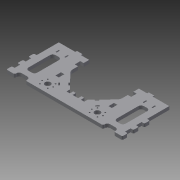
# Autodesk Inventor part: Bulkhead 27021014
Saved by Autodesk Inventor 2015 (Build 190159000, 159)
## iProperties
Created: 2014-06-30
Part Number: Bulkhead 27021014
Material: Generic
Document SubType Name: Modeling
Designer: STACKPOLE
Density: 1 g/cm^3
Appearance: Default
Author: STACKPOLE
Autodesk Inventor part; units mm, degrees
ref_plane "YZ Plane" through (0, 0, 0) normal (1, 0, 0) x (0, 1, 0)
ref_plane "XZ Plane" through (0, 0, 0) normal (0, 1, 0) x (-1, 0, 0)
ref_plane "XY Plane" through (0, 0, 0) normal (0, 0, 1) x (1, 0, 0)
sketch "Sketch1" plane through (0, 0, 0) normal (0, 0, 1) x (1, 0, 0)
  line L0 (0, -90) -> (-103, -90)
  line L1 (0, 0) -> (0, -90) construction
  line L2 (-105, -88) -> (-105, -82)
  line L3 (-103, -80) -> (-100, -80)
  line L4 (-100, -70) -> (-103, -70)
  line L5 (-105, -68) -> (-105, -62)
  line L6 (-103, -60) -> (-100, -60)
  line L7 (-100, -80) -> (-100, -70)
  line L8 (-100, -50) -> (-103, -50)
  line L9 (-105, -48) -> (-105, -42)
  line L10 (-103, -40) -> (-100, -40)
  line L11 (-100, -60) -> (-100, -50)
  line L12 (-100, -40) -> (-100, 0)
  line L13 (-70, 0) -> (-70, 3)
  line L14 (-70, 3) -> (-60, 3)
  line L15 (-60, 3) -> (-60, 0)
  line L16 (-100, 0) -> (-70, 0)
  line L17 (-60, 0) -> (-45, 0)
  line L18 (-45, 0) -> (-45, -29.9568)
  arc A0 (-105, -88) -> (-103, -90) centre (-103, -88) ccw
  arc A1 (-103, -80) -> (-105, -82) centre (-103, -82) ccw
  arc A2 (-105, -68) -> (-103, -70) centre (-103, -68) ccw
  arc A3 (-103, -60) -> (-105, -62) centre (-103, -62) ccw
  arc A4 (-105, -48) -> (-103, -50) centre (-103, -48) ccw
  arc A5 (-103, -40) -> (-105, -42) centre (-103, -42) ccw
  line L19 (0, -90) -> (103, -90)
  line L20 (105, -88) -> (105, -82)
  line L21 (103, -80) -> (100, -80)
  line L22 (100, -70) -> (103, -70)
  line L23 (105, -68) -> (105, -62)
  line L24 (103, -60) -> (100, -60)
  line L25 (100, -80) -> (100, -70)
  line L26 (100, -50) -> (103, -50)
  line L27 (105, -48) -> (105, -42)
  line L28 (103, -40) -> (100, -40)
  line L29 (100, -60) -> (100, -50)
  line L30 (100, -40) -> (100, 0)
  line L31 (70, 0) -> (70, 3)
  line L32 (70, 3) -> (60, 3)
  line L33 (60, 3) -> (60, 0)
  line L34 (100, 0) -> (70, 0)
  line L35 (60, 0) -> (45, 0)
  line L36 (45, 0) -> (45, -29.9568)
  arc A6 (103, -90) -> (105, -88) centre (103, -88) ccw
  arc A7 (105, -82) -> (103, -80) centre (103, -82) ccw
  arc A8 (103, -70) -> (105, -68) centre (103, -68) ccw
  arc A9 (105, -62) -> (103, -60) centre (103, -62) ccw
  arc A10 (103, -50) -> (105, -48) centre (103, -48) ccw
  arc A11 (105, -42) -> (103, -40) centre (103, -42) ccw
  line L37 (-42.1899, -36.907) -> (-16, -64)
  line L38 (16, -64) -> (42.1899, -36.907)
  line L39 (-16, -70) -> (-10, -70)
  line L40 (-10, -70) -> (-10, -64)
  line L41 (-5, -64) -> (-5, -70)
  line L42 (-5, -70) -> (5, -70)
  line L43 (5, -70) -> (5, -64)
  line L44 (10, -64) -> (10, -70)
  line L45 (10, -70) -> (16, -70)
  line L46 (-10, -64) -> (-5, -64)
  line L47 (5, -64) -> (10, -64)
  line L48 (16, -64) -> (16, -70)
  line L49 (-16, -64) -> (-16, -70)
  arc A12 (-45, -29.9568) -> (-42.1899, -36.907) centre (-35, -29.9568) ccw
  arc A13 (42.1899, -36.907) -> (45, -29.9568) centre (35, -29.9568) ccw
  point P0 (-105, -90)
  point P1 (-105, -80)
  point P2 (-105, -70)
  point P3 (-105, -60)
  point P4 (-105, -50)
  point P5 (-105, -40)
  point P6 (105, -90)
  point P7 (105, -80)
  point P8 (105, -70)
  point P9 (105, -60)
  point P10 (105, -50)
  point P11 (105, -40)
  point P12 (-45, -34)
  point P13 (45, -34)
  point P14 (0, -70)
  dimension "d4" = 105
  dimension "d5" = 10
  dimension "d6" = 5
  dimension "d8" = 10
  dimension "d9" = 10
  dimension "d10" = 10
  dimension "d11" = 10
  dimension "d12" = 30
  dimension "d13" = 10
  dimension "d14" = 3
  dimension "d15" = 90
  dimension "d18" = 15
  dimension "d19" = 34
  dimension "d20" = 2
  dimension "d102" = 5
  dimension "d104" = 5
  dimension "d105" = 10
  dimension "d160" = 6
  dimension "d161" = 6
  dimension "d162" = 6
  dimension "d163" = 70
  dimension "d175" = 10
  constraints: 100 end point, 36 symmetric about line, 28 point on circle, 28 point on line, 23 perpendicular, 16 tangent, 14 centre point, 10 parallel, 6 equal radius, 6 horizontal alignment, 5 vertical alignment, 2 horizontal, 1 midpoint, 1 vertical, 6 other
  measures "d4" distance of L0.start point (-105, -90)
  measures "d5" distance of point (-105, -90) point (-105, -80)
  measures "d6" distance of point (-105, -80) L3.end
  measures "d8" distance between parallel lines of L3 L4
  measures "d9" distance of point (-105, -70) point (-105, -60)
  measures "d10" distance between parallel lines of L6 L8
  measures "d11" distance of point (-105, -50) point (-105, -40)
  measures "d12" distance from line of L12 L13.start
  measures "d13" distance of L13.end L14.end
  measures "d14" distance of L13.start L13.end
  measures "d15" distance between parallel lines of L16 L0
  measures "d18" distance of L15.end L17.end
  measures "d19" distance of point (-45, -34) L17.end
  measures "d20" radius of A0
  measures "d102" distance between parallel lines of L41 L40
  measures "d104" distance between parallel lines of L44 L43
  measures "d105" distance between parallel lines of L41 L43
  measures "d160" distance of L37.end L39.start
  measures "d161" distance of L39.start L39.end
  measures "d162" distance of L44.end L45.end
  measures "d163" distance between parallel lines of L35 L42
  measures "d175" radius of A12
extrude "Extrusion1" add sketch "Sketch1" along normal blind 6
sketch "Sketch2" plane through (0, 0, 6) normal (0, 0, 1) x (1, 0, 0)
  line L0 (-103, -90) -> (103, -90) projected
  line L1 (-70, 0) -> (-100, 0) projected
  circle A0 centre (-45, -75) radius 5
  circle A1 centre (-45, -75) radius 10 construction
  line L2 (-45, -75) -> (-52.0711, -67.9289) construction
  line L3 (-45, -75) -> (-55, -75) construction
  line L4 (-55, -75) -> (-45, -75) construction
  circle A2 centre (-52.0711, -67.9289) radius 1.25
  circle A3 centre (-55, -75) radius 1.25
  circle A4 centre (-52.0711, -82.0711) radius 1.25
  line L5 (-45, -65) -> (-45, -85) construction
  circle A5 centre (-37.9289, -67.9289) radius 1.25
  circle A6 centre (-35, -75) radius 1.25
  circle A7 centre (-37.9289, -82.0711) radius 1.25
  line L6 (0, 0) -> (0, -90) construction
  circle A8 centre (45, -75) radius 5
  circle A9 centre (45, -75) radius 10 construction
  line L7 (45, -75) -> (52.0711, -67.9289) construction
  line L8 (45, -75) -> (55, -75) construction
  line L9 (55, -75) -> (45, -75) construction
  circle A10 centre (52.0711, -67.9289) radius 1.25
  circle A11 centre (55, -75) radius 1.25
  circle A12 centre (52.0711, -82.0711) radius 1.25
  line L10 (45, -65) -> (45, -85) construction
  circle A13 centre (37.9289, -67.9289) radius 1.25
  circle A14 centre (35, -75) radius 1.25
  circle A15 centre (37.9289, -82.0711) radius 1.25
  dimension "d23" = 10
  dimension "d25" = 75
  dimension "d26" = 45
  dimension "d27" = 20
  dimension "d28" = 45
  dimension "d29" = 2.5
  dimension "d30" = 2.5
  constraints: 18 end point, 16 centre point, 16 symmetric about line, 8 point on circle, 6 coincident, 1 collinear, 1 midpoint, 1 parallel, 1 perpendicular, 12 other
  measures "d23" diameter of A0
  measures "d25" vertical distance of A0.centre L6.start
  measures "d26" horizontal distance of L6.start A0.centre
  measures "d27" diameter of A1
  measures "d28" angle of L4 L2
  measures "d29" diameter of A2
  measures "d30" diameter of A3
extrude "Extrusion2" cut sketch "Sketch2" against normal blind 6
sketch "Sketch5" plane through (0, 0, 6) normal (0, 0, 1) x (1, 0, 0)
  line L0 (-83, -23) -> (-77, -23)
  line L1 (-72, -28) -> (-72, -67)
  line L2 (-77, -72) -> (-83, -72)
  line L3 (-88, -67) -> (-88, -28)
  line L4 (0, 0) -> (0, -90) construction
  line L5 (83, -23) -> (77, -23)
  line L6 (72, -28) -> (72, -67)
  line L7 (77, -72) -> (83, -72)
  line L8 (88, -67) -> (88, -28)
  arc A0 (-83, -23) -> (-88, -28) centre (-83, -28) ccw
  arc A1 (-72, -28) -> (-77, -23) centre (-77, -28) ccw
  arc A2 (-77, -72) -> (-72, -67) centre (-77, -67) ccw
  arc A3 (-88, -67) -> (-83, -72) centre (-83, -67) ccw
  arc A4 (77, -23) -> (72, -28) centre (77, -28) ccw
  arc A5 (88, -28) -> (83, -23) centre (83, -28) ccw
  arc A6 (83, -72) -> (88, -67) centre (83, -67) ccw
  arc A7 (72, -67) -> (77, -72) centre (77, -67) ccw
  line L9 (-70, 0) -> (-100, 0) projected
  line L10 (-100, 0) -> (-100, -40) projected
  line L11 (-103, -90) -> (103, -90) projected
  point P0 (-88, -23)
  point P1 (-72, -72)
  point P2 (-72, -23)
  point P3 (-88, -72)
  point P4 (88, -23)
  point P5 (72, -72)
  point P6 (72, -23)
  point P7 (88, -72)
  dimension "d65" = 5
  dimension "d187" = 23
  dimension "d188" = 12
  dimension "d189" = 16
  dimension "d190" = 18
  constraints: 18 end point, 16 point on circle, 16 point on line, 16 tangent, 8 centre point, 7 equal radius, 4 symmetric about line, 3 parallel, 1 horizontal, 1 perpendicular
  measures "d65" radius of A0
  measures "d187" distance between parallel lines of L9 L0
  measures "d188" distance between parallel lines of L10 L3
  measures "d189" distance between parallel lines of L1 L3
  measures "d190" distance between parallel lines of L11 L2
extrude "Extrusion5" cut sketch "Sketch5" against normal blind 6
sketch "Sketch3" plane through (0, 0, 6) normal (0, 0, 1) x (1, 0, 0)
  line L0 (-103, -90) -> (103, -90) projected
  line L1 (-70, 0) -> (-100, 0) projected
  line L2 (-88, -12) -> (-86, -12)
  line L3 (-86, -12) -> (-86, -18)
  line L4 (-86, -18) -> (-88, -18)
  line L5 (-88, -18) -> (-88, -12)
  line L6 (-72, -12) -> (-70, -12)
  line L7 (-70, -12) -> (-70, -18)
  line L8 (-70, -18) -> (-72, -18)
  line L9 (-72, -18) -> (-72, -12)
  line L10 (0, 0) -> (0, -90) construction
  line L11 (88, -12) -> (86, -12)
  line L12 (86, -12) -> (86, -18)
  line L13 (86, -18) -> (88, -18)
  line L14 (88, -18) -> (88, -12)
  line L15 (72, -12) -> (70, -12)
  line L16 (70, -12) -> (70, -18)
  line L17 (70, -18) -> (72, -18)
  line L18 (72, -18) -> (72, -12)
  line L19 (-100, 0) -> (-100, -40) projected
  circle A0 centre (-45, -75) radius 5 projected
  line L20 (-16, -64) -> (-42.1899, -36.907) projected
  line L21 (-45, -75) -> (-24.5118, -55.1947) construction
  line L22 (-26.5968, -53.0378) -> (-28.0348, -54.4278)
  line L23 (-28.0348, -54.4278) -> (-23.8647, -58.7417)
  line L24 (-23.8647, -58.7417) -> (-22.4267, -57.3517)
  line L25 (-26.5968, -53.0378) -> (-22.4267, -57.3517)
  line L26 (26.5968, -53.0378) -> (28.0348, -54.4278)
  line L27 (28.0348, -54.4278) -> (23.8647, -58.7417)
  line L28 (23.8647, -58.7417) -> (22.4267, -57.3517)
  line L29 (26.5968, -53.0378) -> (22.4267, -57.3517)
  line L30 (-37.3817, -63.4631) -> (-33.2115, -67.777)
  line L31 (-33.2115, -67.777) -> (-31.7736, -66.387)
  line L32 (-31.7736, -66.387) -> (-35.9437, -62.073)
  line L33 (-35.9437, -62.073) -> (-37.3817, -63.4631)
  line L34 (37.3817, -63.4631) -> (33.2115, -67.777)
  line L35 (33.2115, -67.777) -> (31.7736, -66.387)
  line L36 (31.7736, -66.387) -> (35.9437, -62.073)
  line L37 (35.9437, -62.073) -> (37.3817, -63.4631)
  point P0 (-45, -34)
  dimension "d41" = 6
  dimension "d43" = 12
  dimension "d129" = 12
  dimension "d130" = 14
  dimension "d131" = 2
  dimension "d132" = 2
  dimension "d165" = 3
  dimension "d166" = 3
  dimension "d167" = 2
  dimension "d168" = 11
  dimension "d170" = 2
  dimension "d171" = 3
  dimension "d172" = 3
  constraints: 68 end point, 16 symmetric about line, 7 parallel, 7 perpendicular, 3 point on line, 2 horizontal, 2 horizontal alignment, 1 collinear, 1 midpoint
  measures "d41" distance of L4.end L2.start
  measures "d43" distance between parallel lines of L1 L2
  measures "d129" distance between parallel lines of L5 L19
  measures "d130" distance between parallel lines of L9 L3
  measures "d131" distance of L6.start L6.end
  measures "d132" distance of L2.start L2.end
  measures "d165" distance between parallel lines of L22 L21
  measures "d166" distance between parallel lines of L24 L21
  measures "d167" distance of L22.start L22.end
  measures "d168" distance between parallel lines of L32 L23
  measures "d170" distance of L32.end L30.start
  measures "d171" distance between parallel lines of L33 L21
  measures "d172" distance between parallel lines of L31 L21
sketch "Sketch7" plane through (0, 0, 6) normal (0, 0, 1) x (1, 0, 0)
  line L0 (-100, -70) -> (-100, -80) projected
  line L1 (-103, -90) -> (103, -90) projected
  line L2 (100, -80) -> (100, -70) projected
  line L3 (-90, -90) -> (-70, -90)
  line L4 (-70, -90) -> (-70, -82)
  line L5 (-70, -82) -> (-90, -82)
  line L6 (-90, -82) -> (-90, -90)
  line L7 (90, -90) -> (70, -90)
  line L8 (70, -90) -> (70, -82)
  line L9 (70, -82) -> (90, -82)
  line L10 (90, -82) -> (90, -90)
  point P0 (0, 0)
  dimension "d135" = 10
  dimension "d136" = 8
  dimension "d137" = 20
  dimension "d138" = 10
  dimension "d139" = 20
  dimension "d140" = 8
  constraints: 16 end point, 4 parallel, 2 horizontal, 2 perpendicular, 2 point on line
  measures "d135" distance between parallel lines of L0 L6
  measures "d136" distance of L5.end L3.start
  measures "d137" distance of L4.end L5.end
  measures "d138" distance between parallel lines of L2 L10
  measures "d139" distance of L8.end L9.end
  measures "d140" distance of L9.end L7.start
extrude "Extrusion13" cut sketch "Sketch7" against normal through all
fillet "Fillet4" radius 5 4 edges at (-90, -82, 3) (-70, -82, 3) (70, -82, 3) (90, -82, 3)
fillet "Fillet5" radius 2 4 edges at (-90, -90, 3) (-70, -90, 3) (70, -90, 3) (90, -90, 3)
extrude "Extrusion15" cut sketch "Sketch3" against normal through all contours L2 L3 L4 L5 | L6 L7 L8 L9 | L14 L13 L12 L11 | L18 L17 L16 L15 | L24 L23 L22 L20 | L26 L27 L28 L29 | L33 L32 L31 L30 | L34 L35 L36 L37
fillet "Fillet7" radius 0.5 8 edges at (-26.5968, -53.0378, 3) (-28.0348, -54.4278, 3) (-23.8647, -58.7417, 3) (-22.4267, -57.3517, 3) (26.5968, -53.0378, 3) (28.0348, -54.4278, 3) (23.8647, -58.7417, 3) (22.4267, -57.3517, 3)
sketch "Sketch8" plane through (0, 0, 6) normal (0, 0, 1) x (1, 0, 0)
  line L0 (-45, -29.9568) -> (-45, 0) projected
  line L1 (-45, -10) -> (-51, -10)
  line L2 (-51, -10) -> (-51, -20)
  line L3 (-51, -20) -> (-45, -20)
  line L4 (-45, -20) -> (-45, -10)
  line L5 (-45, 0) -> (-60, 0) projected
  line L6 (-45, -45) -> (-51, -45)
  line L7 (-51, -45) -> (-51, -55)
  line L8 (-51, -55) -> (-45, -55)
  line L9 (-45, -55) -> (-45, -45)
  line L10 (45, 0) -> (45, -29.9568) projected
  line L11 (45, -10) -> (51, -10)
  line L12 (51, -10) -> (51, -20)
  line L13 (51, -20) -> (45, -20)
  line L14 (45, -20) -> (45, -10)
  line L15 (45, -45) -> (51, -45)
  line L16 (51, -45) -> (51, -55)
  line L17 (51, -55) -> (45, -55)
  line L18 (45, -55) -> (45, -45)
  point P0 (0, 0)
  dimension "d177" = 6
  dimension "d178" = 10
  dimension "d179" = 10
  dimension "d180" = 10
  dimension "d181" = 6
  dimension "d182" = 55
  dimension "d183" = 6
  dimension "d184" = 10
  constraints: 32 end point, 8 parallel, 4 horizontal, 4 perpendicular, 3 horizontal alignment, 3 vertical alignment, 2 point on line
  measures "d177" distance of L1.start L1.end
  measures "d178" distance of L1.end L2.end
  measures "d179" distance between parallel lines of L5 L1
  measures "d180" distance of L6.end L7.end
  measures "d181" distance of L7.end L8.end
  measures "d182" distance between parallel lines of L5 L8
  measures "d183" distance of L11.start L11.end
  measures "d184" distance of L11.end L12.end
extrude "Extrusion16" cut sketch "Sketch8" against normal through all
body "Solid1"
